Autodesk Inventor part; units mm, degrees
(part 3 of 3)
sketch "Sketch7" plane through (0, 0, -31.75) normal (0, 0, -1) x (-1, 0, 0)
  line L0 (10.16, -55.8164) -> (-10.16, -55.8164)
  line L1 (-10.16, -55.8164) -> (-10.16, -62.1664)
  line L2 (-10.16, -62.1664) -> (10.16, -62.1664)
  line L3 (10.16, -62.1664) -> (10.16, -55.8164)
  line L4 (12.7, -54.4829) -> (12.7, -63.5) construction
  line L5 (12.7, -58.9914) -> (-12.7, -58.9914) construction
  line L6 (-12.7, -63.5) -> (-12.7, -54.4829) construction
  line L7 (12.7, -63.5) -> (-12.7, -63.5) construction
  line L8 (0, -63.5) -> (0, -58.9914) construction
  point P0 (0, 0)
  dimension "d22" = 6.35
  dimension "d23" = 20.32
  constraints: 12 end point, 4 midpoint, 2 parallel, 1 horizontal, 1 perpendicular, 2 other
  measures "d22" distance of L2.end L0.start
  measures "d23" distance of L0.start L0.end
extrude "Extrusion7" cut sketch "Sketch7" against normal up to surface (6.35 mm away)
pattern_circular "Circular Pattern1" count 4 over 360 about axis through (0, 0, 0) along (0, 0, -1) of "Extrusion7", "Extrusion6", "Extrusion5"
sketch "Sketch12" plane through (-5.0637, -63.5, 0) normal (0, -1, 0) x (1, 0, 0)
  line L0 (17.7637, -31.75) -> (17.7637, -25.4) projected
  line L1 (-7.6363, -31.75) -> (-7.6363, -25.4) projected
  line L2 (17.7637, -31.75) -> (-7.6363, -31.75)
  line L3 (-7.6363, -31.75) -> (-7.6363, -25.4)
  line L4 (-7.6363, -25.4) -> (17.7637, -25.4)
  line L5 (17.7637, -25.4) -> (17.7637, -31.75)
  point P0 (5.0637, 0)
  constraints: 8 end point, 2 parallel, 1 horizontal, 1 perpendicular
extrude "Extrusion10" add sketch "Sketch12" along normal blind 9.525
sketch "Sketch13" plane through (10.16, -62.1664, -31.75) normal (0, 0, -1) x (-1, 0, 0)
  line L0 (0, -2.2543) -> (20.32, -2.2543)
  line L1 (20.32, -2.2543) -> (20.32, -8.6043)
  line L2 (20.32, -8.6043) -> (0, -8.6043)
  line L3 (0, -8.6043) -> (0, -2.2543)
  line L4 (0, 0) -> (0, 6.35) projected
  line L5 (20.32, 6.35) -> (20.32, 0) projected
  line L6 (0, 0) -> (20.32, 0) construction
  line L7 (10.16, 0) -> (10.16, -2.2543) construction
  line L8 (10.16, -8.6043) -> (10.16, -10.8586) construction
  line L9 (22.86, -10.8586) -> (-2.54, -10.8586) construction
  point P0 (10.16, 62.1664)
  dimension "d40" = 6.35
  constraints: 12 end point, 4 midpoint, 3 collinear, 2 parallel, 1 horizontal, 1 perpendicular, 1 point on line
  measures "d40" distance of L0.end L1.end
extrude "Extrusion11" cut sketch "Sketch13" against normal up to surface (6.35 mm away)
sketch "Sketch15" plane through (-5.0637, -73.025, 0) normal (0, -1, 0) x (1, 0, 0)
  circle A0 centre (20.1132, -41.0845) radius 1.778
  circle A1 centre (-9.9858, -41.0845) radius 1.778
  circle A2 centre (-9.9858, -10.9855) radius 1.778
  circle A3 centre (20.1132, -10.9855) radius 1.778
  line L0 (15.2237, -31.75) -> (-5.0963, -31.75) construction
  line L1 (5.0637, -31.75) -> (5.0637, -25.4) construction
  line L2 (-5.0963, -25.4) -> (15.2237, -25.4) construction
  line L3 (-14.6213, -45.72) -> (-14.6213, -6.35) construction
  line L4 (-14.6213, -26.035) -> (24.7487, -26.035) construction
  line L5 (24.7487, -6.35) -> (24.7487, -45.72) construction
  line L6 (23.2882, -44.2595) -> (16.9382, -44.2595)
  line L7 (16.9382, -44.2595) -> (16.9382, -7.8105)
  line L8 (16.9382, -7.8105) -> (23.2882, -7.8105)
  line L9 (23.2882, -7.8105) -> (23.2882, -44.2595)
  line L10 (-13.1608, -44.2595) -> (-6.8108, -44.2595)
  line L11 (-6.8108, -44.2595) -> (-6.8108, -7.8105)
  line L12 (-6.8108, -7.8105) -> (-13.1608, -7.8105)
  line L13 (-13.1608, -7.8105) -> (-13.1608, -44.2595)
  line L14 (16.9382, -31.75) -> (-6.8108, -31.75)
  line L15 (-6.8108, -25.4) -> (16.9382, -25.4)
  line L16 (-7.6363, -31.75) -> (17.7637, -31.75) projected
  line L17 (17.7637, -25.4) -> (-7.6363, -25.4) projected
  point P0 (5.0637, 0)
  dimension "d48" = 3.556
  dimension "d49" = 30.099
  dimension "d50" = 30.099
  dimension "d51" = 3.175
  dimension "d52" = 3.175
  dimension "d53" = 6.35
  dimension "d54" = 3.175
  constraints: 24 end point, 7 symmetric about line, 4 centre point, 4 midpoint, 4 point on line, 3 equal radius, 3 perpendicular, 2 collinear, 2 parallel, 1 horizontal
  measures "d48" diameter of A0
  measures "d49" distance of A1.centre A0.centre
  measures "d50" distance of A3.centre A0.centre
  measures "d51" distance from line of L6 A0.centre
  measures "d52" distance from line of L7 A0.centre
  measures "d53" distance of L6.start L6.end
  measures "d54" distance from line of L8 A3.centre
extrude "Extrusion13" add sketch "Sketch15" against normal blind 3.175
body "Solid1"
